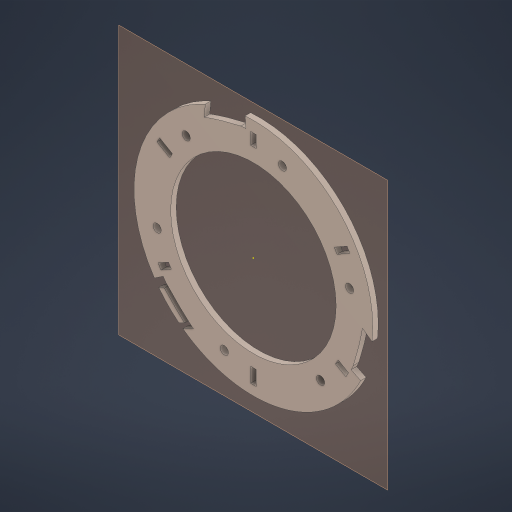
# Autodesk Inventor part: top_centering_ring
Saved by Autodesk Inventor 2023 (Build 270158000, 158)
## iProperties
Created: 2022-06-17
Part Number: top_centering_ring
Material: Generic
Document SubType Name: Modeling
Designer: bananenbrot
Density: 1 g/cm^3
Appearance: Default
Author: bananenbrot
Autodesk Inventor part; units mm, degrees
ref_plane "YZ Plane" through (0, 0, 0) normal (1, 0, 0) x (0, 1, 0)
ref_plane "XZ Plane" through (0, 0, 0) normal (0, 1, 0) x (-1, 0, 0)
ref_plane "XY Plane" through (0, 0, 0) normal (0, 0, 1) x (1, 0, 0)
ref_plane "Work Plane1" through (0, 193.1274, 120) normal (0, 0, 1) x (1, 0, 0)
sketch "Sketch1" plane through (0, 193.1274, 120) normal (0, 0, 1) x (1, 0, 0)
  spline S0 degree 3 poles (-8.5236, -128.7736) (-8.5781, -129.1585) (-8.6317, -129.5435) (-8.7822, -130.6438) (-8.877, -131.3595) (-8.9685, -132.0756) knots 0 0 0 0 0.34999 0.34999 1 1 1 1
  spline S1 degree 3 poles (-8.9685, -132.0756) (-11.4491, -132.616) (-13.9179, -133.213) (-18.9128, -134.5473) (-21.4399, -135.2896) (-23.9457, -136.0968) knots 0.135755 0.135755 0.135755 0.135755 0.897312 0.897312 1.686862 1.686862 1.686862 1.686862
  spline S2 degree 3 poles (-23.9457, -136.0968) (-23.9236, -135.8572) (-23.9012, -135.6176) (-23.8137, -134.697) (-23.7461, -134.0162) (-23.6756, -133.3357) knots 0 0 0 0 0.260219 0.260219 1 1 1 1
  spline S3 degree 3 poles (-23.6756, -133.3357) (-23.6491, -133.1076) (-23.6222, -132.8795) (-23.595, -132.6515) knots 0 0 0 0 1 1 1 1
  spline S4 degree 3 poles (-23.595, -132.6515) (-18.7496, -130.761) (-13.6896, -129.4578) (-8.5236, -128.7736) knots 20.983609 20.983609 20.983609 20.983609 22.549805 22.549805 22.549805 22.549805
  spline S5 degree 3 poles (59.9939, -217.9227) (59.6983, -217.6913) (59.4023, -217.4606) (58.5248, -216.78) (57.9417, -216.3318) (57.3567, -215.8863) knots 0 0 0 0 0.337929 0.337929 1 1 1 1
  spline S6 degree 3 poles (57.3567, -215.8863) (58.129, -213.4679) (58.8464, -211.0314) (60.1883, -206.0385) (60.809, -203.4788) (61.3628, -200.9052) knots 0.135755 0.135755 0.135755 0.135755 0.897312 0.897312 1.686862 1.686862 1.686862 1.686862
  spline S7 degree 3 poles (61.3628, -200.9052) (61.5593, -201.0441) (61.7556, -201.1833) (62.5091, -201.7193) (63.0649, -202.1183) (63.6189, -202.5196) knots 0 0 0 0 0.260219 0.260219 1 1 1 1
  spline S8 degree 3 poles (63.6189, -202.5196) (63.8032, -202.6566) (63.9873, -202.794) (64.1712, -202.9316) knots 0 0 0 0 1 1 1 1
  spline S9 degree 3 poles (64.1712, -202.9316) (63.7306, -205.8156) (63.0951, -208.6728) (61.6213, -213.6722) (60.8623, -215.8215) (59.9939, -217.9227) knots 34.623618 34.623618 34.623618 34.623618 35.502619 35.502619 36.187238 36.187238 36.187238 36.187238
  spline S10 degree 3 poles (-32.5756, -242.7893) (-35.2521, -240.5525) (-37.8465, -238.2164) (-42.8091, -233.429) (-45.1835, -230.9795) (-47.4773, -228.4585) knots 0.183672 0.183672 0.183672 0.183672 1.230026 1.230026 2.252069 2.252069 2.252069 2.252069
  spline S11 degree 3 poles (-47.4773, -228.4585) (-48.486, -228.8718) (-49.4978, -229.2781) (-51.3339, -230.0008) (-52.1579, -230.3199) (-52.9837, -230.6347) knots 0.191156 0.191156 0.191156 0.191156 0.518074 0.518074 0.783091 0.783091 0.783091 0.783091
  spline S12 degree 3 poles (-52.9837, -230.6347) (-54.8569, -227.9885) (-56.5335, -225.1998) (-61.7939, -214.7383) (-64.08, -206.5168) (-65.372, -189.6602) (-64.3656, -181.1864) (-59.1613, -165.1013) (-55.0131, -157.644) (-44.0918, -144.739) (-37.423, -139.4149) (-28.6906, -134.8793) (-27.4411, -134.2804) (-26.1751, -133.7226) knots 9.166621 9.166621 9.166621 9.166621 10.143606 10.143606 12.679507 12.679507 15.215408 15.215408 17.75131 17.75131 20.287211 20.287211 20.703322 20.703322 20.703322 20.703322
  spline S13 degree 3 poles (-26.1751, -133.7226) (-26.2685, -134.6656) (-26.3566, -135.6092) (-26.5417, -137.7293) (-26.6358, -138.907) (-26.7206, -140.0852) knots 0.27267 0.27267 0.27267 0.27267 0.556851 0.556851 0.91105 0.91105 0.91105 0.91105
  spline S14 degree 3 poles (-26.7206, -140.0852) (-23.4453, -138.8857) (-20.1249, -137.8069) (-13.4977, -135.9029) (-10.1891, -135.0714) (-6.8589, -134.3454) knots 0.183672 0.183672 0.183672 0.183672 1.230026 1.230026 2.252069 2.252069 2.252069 2.252069
  spline S15 degree 3 poles (-6.8589, -134.3454) (-6.7126, -133.2651) (-6.5585, -132.1857) (-6.2663, -130.2343) (-6.1307, -129.3611) (-5.9904, -128.4886) knots 0.191156 0.191156 0.191156 0.191156 0.518074 0.518074 0.783091 0.783091 0.783091 0.783091
  spline S16 degree 3 poles (-5.9904, -128.4886) (-5.9303, -128.483) (-5.8702, -128.4775) (2.609, -127.7156) (11.0954, -128.6107) (27.2473, -133.6035) (34.7585, -137.6534) (47.8056, -148.4045) (53.2169, -155.0028) (61.2055, -169.9023) (63.7065, -178.061) (65.044, -191.0327) (65.0284, -195.6223) (64.5336, -200.1615) knots 22.804998 22.804998 22.804998 22.804998 22.823113 22.823113 25.359014 25.359014 27.894915 27.894915 30.430817 30.430817 32.966718 32.966718 34.342971 34.342971 34.342971 34.342971
  spline S17 degree 3 poles (64.5336, -200.1615) (63.7637, -199.6091) (62.9906, -199.0611) (61.247, -197.8407) (60.2742, -197.1704) (59.2962, -196.5078) knots 0.27267 0.27267 0.27267 0.27267 0.556851 0.556851 0.91105 0.91105 0.91105 0.91105
  spline S18 degree 3 poles (59.2962, -196.5078) (58.7011, -199.9229) (57.9804, -203.3168) (56.3185, -210.0089) (55.3791, -213.311) (54.3362, -216.5785) knots 0.183672 0.183672 0.183672 0.183672 1.223566 1.223566 2.252068 2.252068 2.252068 2.252068
  spline S19 degree 3 poles (54.3362, -216.5785) (55.1888, -217.2378) (56.0367, -217.9032) (57.5809, -219.1316) (58.279, -219.6934) (58.9741, -220.259) knots 0.191156 0.191156 0.191156 0.191156 0.514352 0.514352 0.783093 0.783093 0.783093 0.783093
  spline S20 degree 3 poles (-48.3881, -231.4203) (-46.6799, -233.2984) (-44.9285, -235.1379) (-41.2755, -238.7965) (-39.3691, -240.6138) (-37.4172, -242.3803) knots 0.135755 0.135755 0.135755 0.135755 0.897312 0.897312 1.686862 1.686862 1.686862 1.686862
  spline S21 degree 3 poles (-37.4172, -242.3803) (-37.6357, -242.481) (-37.8544, -242.5814) (-38.6954, -242.9659) (-39.3188, -243.2477) (-39.9433, -243.527) knots 0 0 0 0 0.260219 0.260219 1 1 1 1
  spline S22 degree 3 poles (-7.5005, -129.5095) (-7.584, -130.1058) (-7.6655, -130.7024) (-7.8244, -131.8995) (-7.9018, -132.5) (-7.977, -133.1007) knots 0 0 0 0 0.498609 0.498609 1 1 1 1
  spline S23 degree 3 poles (-7.2694, -129.468) (-7.3079, -129.4749) (-7.3464, -129.4818) (-7.4234, -129.4956) (-7.4619, -129.5026) (-7.5005, -129.5095) knots 0 0 0 0 0.500065 0.500065 1 1 1 1
  spline S24 degree 3 poles (-7.8342, -133.3176) (-7.745, -132.6733) (-7.6532, -132.0292) (-7.4648, -130.7461) (-7.3683, -130.1068) (-7.2694, -129.468) knots 0 0 0 0 0.50156 0.50156 1 1 1 1
  spline S25 degree 3 poles (-25.4683, -138.246) (-22.5608, -137.2415) (-19.6212, -136.3286) (-13.7391, -134.691) (-10.7949, -133.9632) (-7.8342, -133.3176) knots -1.831866 -1.831866 -1.831866 -1.831866 -0.909091 -0.909091 0 0 0 0
  spline S26 degree 3 poles (-24.8602, -131.8333) (-24.9726, -132.8737) (-25.0786, -133.9151) (-25.2822, -136.0525) (-25.3792, -137.149) (-25.4683, -138.246) knots -0.64407 -0.64407 -0.64407 -0.64407 -0.330168 -0.330168 0 0 0 0
  spline S27 degree 3 poles (-40.8735, -245.1308) (-42.2164, -244.0754) (-43.5199, -242.9667) (-51.1195, -235.9758) (-56.2587, -228.9623) (-63.5596, -213.3602) (-65.6514, -204.9207) (-66.4822, -187.715) (-65.2134, -179.1132) (-59.4499, -162.8802) (-55.0103, -155.4042) (-43.5155, -142.5746) (-36.5701, -137.3438) (-27.5163, -132.9614) (-26.1964, -132.3752) (-24.8602, -131.8333) knots -34.104259 -34.104259 -34.104259 -34.104259 -33.590314 -33.590314 -31.006444 -31.006444 -28.422574 -28.422574 -25.838703 -25.838703 -23.254833 -23.254833 -20.670963 -20.670963 -20.237237 -20.237237 -20.237237 -20.237237
  spline S28 degree 3 poles (-39.0691, -244.3542) (-39.3864, -244.4922) (-39.704, -244.6296) (-40.3055, -244.8884) (-40.5894, -245.0099) (-40.8735, -245.1308) knots 0 0 0 0 0.528438 0.528438 1 1 1 1
  spline S29 degree 3 poles (-35.2346, -242.5871) (-35.8743, -242.8888) (-36.5154, -243.1876) (-37.7935, -243.7765) (-38.4307, -244.0667) (-39.0691, -244.3542) knots 0 0 0 0 0.502528 0.502528 1 1 1 1
  spline S30 degree 3 poles (-47.9961, -230.049) (-46.0008, -232.2434) (-43.9453, -234.3847) (-39.6934, -238.5693) (-37.494, -240.6129) (-35.2346, -242.5871) knots -1.789969 -1.789969 -1.789969 -1.789969 -0.90011 -0.90011 0 0 0 0
  spline S31 degree 3 poles (-51.3445, -231.432) (-50.7863, -231.2062) (-50.2289, -230.9784) (-49.1128, -230.5175) (-48.554, -230.2843) (-47.9961, -230.049) knots 0 0 0 0 0.498609 0.498609 1 1 1 1
  spline S32 degree 3 poles (-51.496, -231.2526) (-51.4708, -231.2825) (-51.4455, -231.3124) (-51.395, -231.3722) (-51.3698, -231.4021) (-51.3445, -231.432) knots 0 0 0 0 0.500065 0.500065 1 1 1 1
  spline S33 degree 3 poles (-47.8797, -229.817) (-48.4823, -230.0619) (-49.086, -230.3044) (-50.2914, -230.7828) (-50.8933, -231.0189) (-51.496, -231.2526) knots 0 0 0 0 0.50156 0.50156 1 1 1 1
  spline S34 degree 3 poles (-34.7946, -242.6244) (-37.1182, -240.6086) (-39.3786, -238.5193) (-43.7379, -234.2441) (-45.8403, -232.0583) (-47.8797, -229.817) knots -1.831866 -1.831866 -1.831866 -1.831866 -0.909091 -0.909091 0 0 0 0
  spline S35 degree 3 poles (-40.6522, -245.304) (-39.695, -244.8812) (-38.7401, -244.4523) (-36.7872, -243.5599) (-35.7891, -243.0956) (-34.7946, -242.6244) knots -0.64407 -0.64407 -0.64407 -0.64407 -0.330168 -0.330168 0 0 0 0
  spline S36 degree 3 poles (0, -259.2712) (-7.8255, -259.2712) (-15.5958, -257.8824) (-29.3299, -252.8022) (-35.3004, -249.4738) (-40.6522, -245.304) knots -38.525501 -38.525501 -38.525501 -38.525501 -36.174184 -36.174184 -34.13245 -34.13245 -34.13245 -34.13245
  spline S37 degree 3 poles (65.473, -202.5232) (64.9341, -206.2791) (64.0716, -209.9903) (60.2232, -221.8041) (55.9814, -229.3941) (44.8272, -242.5208) (38.0214, -247.9321) (30.3701, -251.8868) (26.0379, -254.1258) (21.4715, -255.879) (12.0364, -258.3494) (7.1967, -259.0591) (1.5485, -259.2576) (0.774, -259.2712) (0, -259.2712) knots -6.311327 -6.311327 -6.311327 -6.311327 -5.167741 -5.167741 -2.58387 -2.58387 0 0 0 1.462965 1.462965 2.925931 2.925931 3.158484 3.158484 3.158484 3.158484
  spline S38 degree 3 poles (63.8982, -201.3489) (64.1764, -201.5546) (64.4542, -201.761) (64.9791, -202.1525) (65.2262, -202.3377) (65.473, -202.5232) knots 0 0 0 0 0.528438 0.528438 1 1 1 1
  spline S39 degree 3 poles (60.4507, -198.9117) (61.0317, -199.3148) (61.6111, -199.7206) (62.7601, -200.5331) (63.3301, -200.9398) (63.8982, -201.3489) knots 0 0 0 0 0.502528 0.502528 1 1 1 1
  spline S40 degree 3 poles (55.9731, -216.2325) (56.8758, -213.4073) (57.7025, -210.5565) (59.2006, -204.782) (59.8706, -201.8554) (60.4507, -198.9117) knots -1.789969 -1.789969 -1.789969 -1.789969 -0.90011 -0.90011 0 0 0 0
  spline S41 degree 3 poles (58.8449, -218.4408) (58.3703, -218.0703) (57.8944, -217.7014) (56.9372, -216.9653) (56.4558, -216.598) (55.9731, -216.2325) knots 0 0 0 0 0.498609 0.498609 1 1 1 1
  spline S42 degree 3 poles (58.7654, -218.6617) (58.7787, -218.6248) (58.7919, -218.5881) (58.8184, -218.5145) (58.8317, -218.4776) (58.8449, -218.4408) knots 0 0 0 0 0.500065 0.500065 1 1 1 1
  spline S43 degree 3 poles (55.7139, -216.2477) (56.2274, -216.6471) (56.7392, -217.0487) (57.7563, -217.8534) (58.2616, -218.2566) (58.7654, -218.6617) knots 0 0 0 0 0.50156 0.50156 1 1 1 1
  spline S44 degree 3 poles (60.2629, -198.512) (59.679, -201.5321) (58.9999, -204.5344) (57.477, -210.4472) (56.6352, -213.3609) (55.7139, -216.2477) knots -1.831866 -1.831866 -1.831866 -1.831866 -0.909091 -0.909091 0 0 0 0
  spline S45 degree 3 poles (65.5124, -202.245) (64.6675, -201.6274) (63.8187, -201.0149) (62.0694, -199.7698) (61.1683, -199.1376) (60.2629, -198.512) knots -0.64407 -0.64407 -0.64407 -0.64407 -0.330168 -0.330168 0 0 0 0
  spline S46 degree 3 poles (-24.5995, -131.7282) (-18.0519, -129.1049) (-11.117, -127.542) (4.5396, -126.5799) (13.1572, -127.7358) (29.4645, -133.2858) (36.9981, -137.6268) (49.9774, -148.9523) (55.2989, -155.8285) (63.0067, -171.2336) (65.3193, -179.6153) (66.3106, -192.8981) (66.1582, -197.6047) (65.5124, -202.245) knots -20.209057 -20.209057 -20.209057 -20.209057 -18.087092 -18.087092 -15.503222 -15.503222 -12.919352 -12.919352 -10.335481 -10.335481 -7.751611 -7.751611 -6.339562 -6.339562 -6.339562 -6.339562
  spline S47 degree 3 poles (-24.8291, -133.6792) (-24.79, -133.3354) (-24.7502, -132.9917) (-24.6736, -132.3413) (-24.6368, -132.0347) (-24.5995, -131.7282) knots 0 0 0 0 0.528438 0.528438 1 1 1 1
  spline S48 degree 3 poles (-25.216, -137.8835) (-25.1575, -137.1787) (-25.0957, -136.4741) (-24.9666, -135.0727) (-24.8993, -134.3758) (-24.8291, -133.6792) knots 0 0 0 0 0.502528 0.502528 1 1 1 1
  spline S49 degree 3 poles (-7.977, -133.1007) (-10.875, -133.7316) (-13.7572, -134.4411) (-19.5071, -136.031) (-22.3766, -136.914) (-25.216, -137.8835) knots -1.789969 -1.789969 -1.789969 -1.789969 -0.90011 -0.90011 0 0 0 0
  circle A0 centre (0, -193.1274) radius 45
  line L0 (44.0013, -165.9912) -> (50.9295, -161.9912)
  line L1 (52.4295, -164.5893) -> (50.9295, -161.9912)
  line L2 (52.4295, -164.5893) -> (45.5013, -168.5893)
  line L3 (44.0013, -165.9912) -> (45.5013, -168.5893)
  line L4 (-50.9295, -161.9912) -> (-44.0013, -165.9912)
  line L5 (-50.9295, -161.9912) -> (-52.4295, -164.5893)
  line L6 (-45.5013, -168.5893) -> (-52.4295, -164.5893)
  line L7 (-45.5013, -168.5893) -> (-44.0013, -165.9912)
  line L8 (-1.5, -252.8018) -> (-1.5, -244.8018)
  line L9 (1.5, -244.8018) -> (-1.5, -244.8018)
  line L10 (1.5, -244.8018) -> (1.5, -252.8018)
  line L11 (-1.5, -252.8018) -> (1.5, -252.8018)
  spline S50 degree 3 poles (-38.3585, -245.4981) (-37.4952, -245.1076) (-36.634, -244.712) (-34.7053, -243.8123) (-33.6384, -243.3049) (-32.5756, -242.7893) knots 0.27267 0.27267 0.27267 0.27267 0.556851 0.556851 0.91105 0.91105 0.91105 0.91105
  spline S51 degree 3 poles (58.9741, -220.259) (56.7613, -225.0687) (53.9634, -229.6006) (47.641, -237.4817) (44.2425, -240.8723) (36.7621, -246.8445) (32.7031, -249.4078) (28.3993, -251.5016) (20.7982, -255.1996) (12.5473, -257.3776) (4.1113, -257.9129) (-4.3247, -258.4483) (-12.7847, -257.3308) (-27.0897, -252.4941) (-33.0126, -249.4137) (-38.3585, -245.4981) knots 36.443216 36.443216 36.443216 36.443216 38.038521 38.038521 39.474327 39.474327 40.910133 40.910133 40.910133 43.446034 43.446034 43.446034 45.981935 45.981935 47.976198 47.976198 47.976198 47.976198
  spline S52 degree 3 poles (-40.5762, -243.7993) (-41.2556, -243.2553) (-41.9245, -242.6972) (-45.8604, -239.2766) (-48.8363, -236.1131) (-51.4702, -232.686) knots 7.346153 7.346153 7.346153 7.346153 7.607704 7.607704 8.910509 8.910509 8.910509 8.910509
  spline S53 degree 3 poles (-51.4702, -232.686) (-51.1097, -232.5407) (-50.7495, -232.3946) (-49.7213, -231.9749) (-49.0541, -231.6991) (-48.3881, -231.4203) knots 0 0 0 0 0.34999 0.34999 1 1 1 1
  spline S54 degree 3 poles (-39.9433, -243.527) (-40.1542, -243.618) (-40.3651, -243.7088) (-40.5762, -243.7993) knots 0 0 0 0 1 1 1 1
  point P0 (4.1113, -257.9129)
  dimension "d0" = 90
  constraints: 1 centre point, 1 coincident
  measures "d0" diameter of A0
extrude "Extrusion1" add sketch "Sketch1" against normal blind 3 contours S10 S11 S12 S13 S14 S15 S16 S17 S18 S19 S51 S50 | S20 S21 S54 S52 S53
sketch "Sketch2" plane through (0, 193.1274, 120) normal (0, 0, 1) x (1, 0, 0)
  point P0 (0, -193.1274)
sketch "Sketch3" plane through (0, 193.1274, 120) normal (0, 0, 1) x (1, 0, 0)
  ellipse E0 centre (-53.6671, -215.1652) end of major axis (-140.5176, -322.1703) minor radius 96.9651 (54.3362, -216.5785) -> (59.2962, -196.5078) ccw projected
  ellipse E1 centre (-0.0025, -193.1242) end of major axis (40.4209, -243.9233) minor radius 64.9177 (4.1113, -257.9129) -> (58.9741, -220.259) ccw projected
  circle A0 centre (-0.0025, -193.1242) radius 59.1844
  line L0 (58.3315, -221.6144) -> (53.1782, -219.0975)
  spline S0 degree 3 poles (54.3362, -216.5785) (55.1888, -217.2378) (56.0367, -217.9032) (57.5809, -219.1316) (58.279, -219.6934) (58.9741, -220.259) knots 0.191156 0.191156 0.191156 0.191156 0.514352 0.514352 0.783093 0.783093 0.783093 0.783093 projected
  point P0 (0, -193.1274)
  dimension "d3" = 1.5
  constraints: 2 end point, 2 point on circle, 1 centre point, 1 coincident, 1 line through centre, 3 other
  measures "d3" distance of point (58.974, -220.259) L0.start
extrude "Extrusion2" cut sketch "Sketch3" against normal blind 3 contours S0 E1 L0 A0
pattern_circular "Circular Pattern1" count 3 over 360 about axis through (0, 0, 120) along (0, 0, -1) of "Extrusion2"
sketch "Sketch4" plane through (0, 193.1274, 120) normal (0, 0, 1) x (1, 0, 0)
  line L0 (46.1583, -218.0449) -> (44.6583, -220.6429) projected
  line L1 (50.2726, -223.8844) -> (44.6583, -220.6429) projected
  line L2 (50.2726, -223.8844) -> (51.7726, -221.2863) projected
  line L3 (46.1583, -218.0449) -> (51.7726, -221.2863) projected
  line L4 (-44.6583, -220.6429) -> (-46.1583, -218.0449) projected
  line L5 (-51.7726, -221.2863) -> (-46.1583, -218.0449) projected
  line L6 (-51.7726, -221.2863) -> (-50.2726, -223.8844) projected
  line L7 (-44.6583, -220.6429) -> (-50.2726, -223.8844) projected
  arc A0 (-4.0983, -134.0887) -> (-6.8589, -134.3454) centre (-0.0015, -193.1312) ccw projected
  ellipse E0 centre (45.933, -228.6071) end of major axis (182.0447, -250.3428) minor radius 96.9844 (-6.8589, -134.3454) -> (-26.7206, -140.0852) ccw projected
  ellipse E1 centre (3482.2315, 3108.1321) end of major axis (6968.4661, 6441.6093) minor radius 583.7417 (-26.1751, -133.7226) -> (-26.7206, -140.0852) ccw projected
  line L8 (-53.8361, -229.4005) -> (-49.0799, -226.1961) projected
  arc A1 (-49.0799, -226.1961) -> (-47.4773, -228.4585) centre (0.004, -193.1268) ccw projected
  ellipse E2 centre (7.7598, -135.6085) end of major axis (56.992, -264.3525) minor radius 96.9844 (-47.4773, -228.4585) -> (-32.5756, -242.7893) ccw projected
  ellipse E3 centre (-4600.0924, 1171.9444) end of major axis (29.9029, -180.4853) minor radius 583.7419 (-38.3585, -245.4981) -> (-32.5756, -242.7893) ccw projected
  line L9 (58.3315, -221.6144) -> (53.1782, -219.0975) projected
  arc A2 (53.1782, -219.0975) -> (54.3362, -216.5785) centre (-0.0025, -193.1242) ccw projected
  ellipse E4 centre (-53.6671, -215.1652) end of major axis (-140.5176, -322.1703) minor radius 96.9651 (54.3362, -216.5785) -> (59.2962, -196.5078) ccw projected
  ellipse E5 centre (1117.8591, -4859.4595) end of major axis (-25.8998, -173.5519) minor radius 583.7418 (64.5336, -200.1615) -> (59.2962, -196.5078) ccw projected
  line L10 (-4.4953, -128.3674) -> (-4.0983, -134.0887) projected
  circle A3 centre (0, -193.1274) radius 45 projected
  line L11 (52.4295, -164.5893) -> (45.5013, -168.5893) projected
  line L12 (45.5013, -168.5893) -> (44.0013, -165.9912) projected
  line L13 (44.0013, -165.9912) -> (50.9295, -161.9912) projected
  line L14 (50.9295, -161.9912) -> (52.4295, -164.5893) projected
  line L15 (-45.5013, -168.5893) -> (-52.4295, -164.5893) projected
  line L16 (-52.4295, -164.5893) -> (-50.9295, -161.9912) projected
  line L17 (-50.9295, -161.9912) -> (-44.0013, -165.9912) projected
  line L18 (-44.0013, -165.9912) -> (-45.5013, -168.5893) projected
  line L19 (1.5, -244.8018) -> (1.5, -252.8018) projected
  line L20 (1.5, -252.8018) -> (-1.5, -252.8018) projected
  line L21 (-1.5, -252.8018) -> (-1.5, -244.8018) projected
  line L22 (-1.5, -244.8018) -> (1.5, -244.8018) projected
  line L23 (-1.5, -140.6945) -> (1.5, -140.6945) projected
  line L24 (1.5, -134.2116) -> (1.5, -140.6945) projected
  line L25 (1.5, -134.2116) -> (-1.5, -134.2116) projected
  line L26 (-1.5, -140.6945) -> (-1.5, -134.2116) projected
  constraints: 9 other
extrude "Extrusion3" cut sketch "Sketch4" against normal blind 10 contours L3 L2 L1 L0 | L7 L6 L5 L4 | L26 L25 L24 L23
sketch "Sketch5" plane through (0, 193.1274, 120) normal (0, 0, 1) x (1, 0, 0)
  circle A0 centre (0, -193.1274) radius 45 projected
  circle A1 centre (-36.5231, -153.7993) radius 2.25
  dimension "d11" = 4.5
  constraints: 1 centre point, 1 other
  measures "d11" diameter of A1
extrude "Extrusion4" cut sketch "Sketch5" against normal blind 10 contours A1
pattern_circular "Circular Pattern2" count 6 over 360 about axis through (0, 0, -10) along (0, 0, 1) of "Extrusion4"
body "Solid1"
